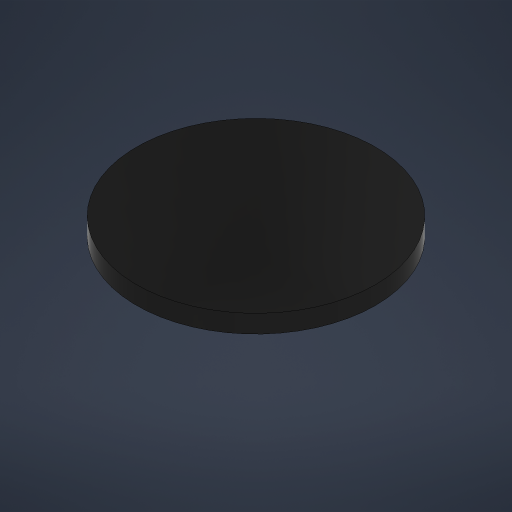
# Autodesk Inventor part: COne_mirror
Saved by Autodesk Inventor 2024.2 (Build 282272000, 272)
## iProperties
Created: 2024-02-16
Part Number: COne_mirror
Material: 一般
Document SubType Name: Modeling
Designer: Hanaoka
Density: 1 g/cm^3
Appearance: 滑らか - 黒
Author: Hanaoka
Autodesk Inventor part; units mm, degrees
ref_plane "YZ Plane" through (0, 0, 0) normal (1, 0, 0) x (0, 1, 0)
ref_plane "XZ Plane" through (0, 0, 0) normal (0, 1, 0) x (-1, 0, 0)
ref_plane "XY Plane" through (0, 0, 0) normal (0, 0, 1) x (1, 0, 0)
sketch "スケッチ1" plane through (0, 0, 0) normal (0, 0, 1) x (1, 0, 0)
  line L0 (5, 2.8868) -> (22.5, 12.9904)
  line L1 (22.5, 12.9904) -> (-22.5, 12.9904)
  line L2 (-22.5, 12.9904) -> (-5, 2.8868)
  line L3 (-22.5, 12.9904) -> (-22.5, 14.9904)
  line L4 (-22.5, 14.9904) -> (-25, 14.9904)
  line L5 (-25, 14.9904) -> (-25, 12.9904)
  line L6 (-25, 12.9904) -> (-26.5, 12.9904)
  line L7 (-26.5, 12.9904) -> (-26.5, 16.9904)
  line L8 (-26.5, 16.9904) -> (26.5, 16.9904)
  line L9 (26.5, 16.9904) -> (26.5, 12.9904)
  line L10 (26.5, 12.9904) -> (25, 12.9904)
  line L11 (25, 12.9904) -> (25, 14.9904)
  line L12 (25, 14.9904) -> (22.5, 14.9904)
  line L13 (22.5, 14.9904) -> (22.5, 12.9904)
  line L14 (-22.5, 14.9904) -> (-22.5, 54.9904)
  line L15 (-22.5, 54.9904) -> (22.5, 54.9904)
  line L16 (22.5, 54.9904) -> (22.5, 14.9904)
  arc A0 (-5, 2.8868) -> (5, 2.8868) centre (0, 11.547) ccw
  line L17 (0, 0) -> (0, 54.9904)
  line L18 (-25, 12.9904) -> (-25, 4.9904)
  line L19 (-25, 4.9904) -> (-26.5, 4.9904)
  line L20 (-26.5, 4.9904) -> (-26.5, 12.9904)
  line L21 (25, 12.9904) -> (25, 4.9904)
  line L22 (25, 4.9904) -> (26.5, 4.9904)
  line L23 (26.5, 4.9904) -> (26.5, 12.9904)
  point P0 (0, 1.547)
  point P1 (0, 16.9904)
  dimension "d0" = 45
  dimension "d1" = 30
  dimension "d2" = 2.5
  dimension "d3" = 1.5
  dimension "d4" = 2
  dimension "d5" = 4
  dimension "d6" = 40
  dimension "d7" = 10
  dimension "d9" = 8
  dimension "d10" = 50
  constraints: 48 end point, 12 perpendicular, 9 equal length, 4 point on line, 3 vertical, 2 point on circle, 2 tangent, 1 centre point, 1 collinear, 1 horizontal, 1 midpoint
  measures "d0" distance of L0.end L1.end
  measures "d1" angle of L0 L1
  measures "d2" distance of L3.end L4.end
  measures "d3" distance of L5.end L6.end
  measures "d4" distance of L1.end L3.end
  measures "d5" distance of L6.end L7.end
  measures "d6" distance of L15.end L12.end
  measures "d7" radius of A0
  measures "d9" distance of L19.end L6.end
  measures "d10" distance of L21.end L18.end
revolve "回転1" add sketch "スケッチ1" angle 360 about axis through (0, 0, 0) along (0, 1, 0) contours A0 L17 L1 L0 | L1 L17 L8 L16 L13 | L16 L8 L9 L10 L11 L12
fillet "フィレット1" radius 1 2 edges at (-25, 12.9904, 0) (-22.5, 12.9904, 0)
